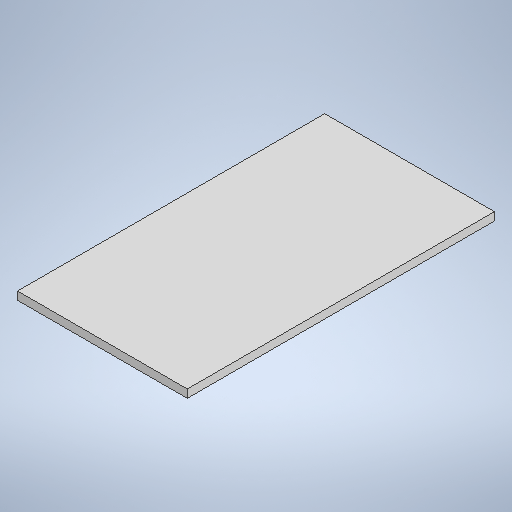
# Autodesk Inventor part: tatakan_mcu
Saved by Autodesk Inventor 2025.2 (Build 292293000, 293)
## iProperties
Created: 2025-02-18
Part Number: tatakan_mcu
Material: Generic
Document SubType Name: Modeling
Designer: ACER
Density: 1 g/cm^3
Appearance: Default
Author: ACER
Autodesk Inventor part; units mm, degrees
ref_plane "YZ Plane" through (0, 0, 0) normal (1, 0, 0) x (0, 1, 0)
ref_plane "XZ Plane" through (0, 0, 0) normal (0, 1, 0) x (-1, 0, 0)
ref_plane "XY Plane" through (0, 0, 0) normal (0, 0, 1) x (1, 0, 0)
sketch "Sketch1" plane through (0, 0, 0) normal (0, 1, 0) x (-1, 0, 0)
  line L0 (-21, 38) -> (21, 38)
  line L1 (21, 38) -> (21, -38)
  line L2 (21, -38) -> (-21, -38)
  line L3 (-21, -38) -> (-21, 38)
  line L4 (-21, 38) -> (21, -38) construction
  line L5 (21, 38) -> (-21, -38) construction
  point P0 (0, 0)
  dimension "d0" = 76
  dimension "d1" = 42
  constraints: 12 end point, 2 midpoint, 2 parallel, 1 horizontal, 1 perpendicular
  measures "d0" distance of L0.end L1.end
  measures "d1" distance of L1.end L2.end
extrude "Extrusion1" add sketch "Sketch1" along normal blind 2
body "Solid1"
